Autodesk Inventor part; units mm, degrees
(part 8 of 11)
  line L1498 (15.1661, 13.0288) -> (15.4178, 12.4694)
  arc A2998 (15.3831, 12.4537) -> (15.4526, 12.485) centre (15.4178, 12.4694) ccw
  arc A2999 (15.2008, 13.0444) -> (15.1314, 13.0131) centre (15.1661, 13.0288) ccw
  line L1499 (15.4178, 12.4694) -> (15.6004, 11.8837)
  arc A3000 (15.5641, 11.8724) -> (15.6368, 11.8951) centre (15.6004, 11.8837) ccw
  arc A3001 (15.4542, 12.4807) -> (15.3815, 12.458) centre (15.4178, 12.4694) ccw
  line L1500 (15.6004, 11.8837) -> (15.7112, 11.2804)
  arc A3002 (15.6737, 11.2735) -> (15.7486, 11.2872) centre (15.7112, 11.2804) ccw
  arc A3003 (15.6379, 11.8906) -> (15.5629, 11.8769) centre (15.6004, 11.8837) ccw
  line L1501 (15.7112, 11.2804) -> (15.748, 10.668)
  arc A3004 (15.71, 10.6657) -> (15.786, 10.6703) centre (15.748, 10.668) ccw
  arc A3005 (15.7492, 11.2827) -> (15.6731, 11.2781) centre (15.7112, 11.2804) ccw
  line L1502 (15.748, 10.668) -> (15.6894, 10.0106)
  arc A3006 (15.6514, 10.014) -> (15.7273, 10.0072) centre (15.6894, 10.0106) ccw
  arc A3007 (15.7859, 10.6646) -> (15.71, 10.6714) centre (15.748, 10.668) ccw
  line L1503 (15.6894, 10.0106) -> (15.5482, 9.3659)
  arc A3008 (15.511, 9.3741) -> (15.5854, 9.3578) centre (15.5482, 9.3659) ccw
  arc A3009 (15.7266, 10.0025) -> (15.6522, 10.0188) centre (15.6894, 10.0106) ccw
  line L1504 (15.5482, 9.3659) -> (15.3268, 8.7442)
  arc A3010 (15.2909, 8.757) -> (15.3626, 8.7314) centre (15.3268, 8.7442) ccw
  arc A3011 (15.5841, 9.3532) -> (15.5123, 9.3787) centre (15.5482, 9.3659) ccw
  line L1505 (15.3268, 8.7442) -> (15.0285, 8.1555)
  arc A3012 (14.9945, 8.1727) -> (15.0625, 8.1383) centre (15.0285, 8.1555) ccw
  arc A3013 (15.3607, 8.727) -> (15.2928, 8.7614) centre (15.3268, 8.7442) ccw
  line L1506 (15.0285, 8.1555) -> (14.6584, 7.6091)
  arc A3014 (14.6268, 7.6305) -> (14.6899, 7.5877) centre (14.6584, 7.6091) ccw
  arc A3015 (15.0601, 8.1341) -> (14.997, 8.1768) centre (15.0285, 8.1555) ccw
  line L1507 (14.6584, 7.6091) -> (14.2222, 7.1138)
  arc A3016 (14.1936, 7.139) -> (14.2507, 7.0887) centre (14.2222, 7.1138) ccw
  arc A3017 (14.687, 7.5839) -> (14.6298, 7.6343) centre (14.6584, 7.6091) ccw
  line L1508 (14.2222, 7.1138) -> (13.7269, 6.6776)
  arc A3018 (13.7017, 6.7062) -> (13.7521, 6.649) centre (13.7269, 6.6776) ccw
  arc A3019 (14.2473, 7.0853) -> (14.197, 7.1424) centre (14.2222, 7.1138) ccw
  line L1509 (13.7269, 6.6776) -> (13.1805, 6.3075)
  arc A3020 (13.1592, 6.339) -> (13.2019, 6.2759) centre (13.1805, 6.3075) ccw
  arc A3021 (13.7483, 6.6461) -> (13.7055, 6.7092) centre (13.7269, 6.6776) ccw
  line L1510 (13.1805, 6.3075) -> (12.5917, 6.0093)
  arc A3022 (12.5745, 6.0433) -> (12.609, 5.9753) centre (12.5917, 6.0093) ccw
  arc A3023 (13.1977, 6.2735) -> (13.1633, 6.3415) centre (13.1805, 6.3075) ccw
  line L1511 (12.5917, 6.0093) -> (11.97, 5.7878)
  arc A3024 (11.9573, 5.8237) -> (11.9828, 5.7519) centre (11.97, 5.7878) ccw
  arc A3025 (12.6045, 5.9734) -> (12.579, 6.0452) centre (12.5917, 6.0093) ccw
  line L1512 (11.97, 5.7878) -> (11.3254, 5.6466)
  arc A3026 (11.3172, 5.6838) -> (11.3335, 5.6094) centre (11.3254, 5.6466) ccw
  arc A3027 (11.9782, 5.7506) -> (11.9619, 5.825) centre (11.97, 5.7878) ccw
  line L1513 (11.3254, 5.6466) -> (10.668, 5.588)
  arc A3028 (10.6646, 5.626) -> (10.6714, 5.5501) centre (10.668, 5.588) ccw
  arc A3029 (11.3288, 5.6087) -> (11.322, 5.6846) centre (11.3254, 5.6466) ccw
  line L1514 (10.668, 5.588) -> (10.668, 6.858)
  arc A3030 (10.7061, 6.858) -> (10.6299, 6.858) centre (10.668, 6.858) ccw
  arc A3031 (10.6299, 5.588) -> (10.7061, 5.588) centre (10.668, 5.588) ccw
  line L1515 (10.668, 6.858) -> (11.1934, 6.8774)
  arc A3032 (11.1948, 6.8393) -> (11.192, 6.9155) centre (11.1934, 6.8774) ccw
  arc A3033 (10.6666, 6.8961) -> (10.6694, 6.8199) centre (10.668, 6.858) ccw
  line L1516 (11.1934, 6.8774) -> (11.7108, 6.9714)
  arc A3034 (11.7176, 6.9339) -> (11.704, 7.0089) centre (11.7108, 6.9714) ccw
  arc A3035 (11.1866, 6.9149) -> (11.2003, 6.8399) centre (11.1934, 6.8774) ccw
  line L1517 (11.7108, 6.9714) -> (12.2094, 7.1381)
  arc A3036 (12.2215, 7.1019) -> (12.1974, 7.1742) centre (12.2094, 7.1381) ccw
  arc A3037 (11.6987, 7.0075) -> (11.7228, 6.9353) centre (11.7108, 6.9714) ccw
  line L1518 (12.2094, 7.1381) -> (12.6793, 7.374)
  arc A3038 (12.6964, 7.34) -> (12.6623, 7.4081) centre (12.6794, 7.374) ccw
  arc A3039 (12.1924, 7.1721) -> (12.2265, 7.104) centre (12.2094, 7.1381) ccw
  line L1519 (12.6793, 7.374) -> (13.1109, 7.6744)
  arc A3040 (13.1326, 7.6431) -> (13.0891, 7.7057) centre (13.1109, 7.6744) ccw
  arc A3041 (12.6576, 7.4053) -> (12.7011, 7.3427) centre (12.6793, 7.374) ccw
  line L1520 (13.1109, 7.6744) -> (13.4952, 8.0332)
  arc A3042 (13.5212, 8.0053) -> (13.4693, 8.061) centre (13.4952, 8.0332) ccw
  arc A3043 (13.0849, 7.7023) -> (13.1369, 7.6465) centre (13.1109, 7.6744) ccw
  line L1521 (13.4952, 8.0332) -> (13.8247, 8.443)
  arc A3044 (13.8544, 8.4191) -> (13.795, 8.4669) centre (13.8247, 8.443) ccw
  arc A3045 (13.4655, 8.057) -> (13.5249, 8.0093) centre (13.4952, 8.0332) ccw
  line L1522 (13.8247, 8.443) -> (14.0924, 8.8955)
  arc A3046 (14.1252, 8.8761) -> (14.0596, 8.9149) centre (14.0924, 8.8955) ccw
  arc A3047 (13.7919, 8.4624) -> (13.8575, 8.4236) centre (13.8247, 8.443) ccw
  line L1523 (14.0924, 8.8955) -> (14.293, 9.3815)
  arc A3048 (14.3282, 9.367) -> (14.2578, 9.3961) centre (14.293, 9.3815) ccw
  arc A3049 (14.0572, 8.91) -> (14.1276, 8.881) centre (14.0924, 8.8955) ccw
  line L1524 (14.293, 9.3815) -> (14.4224, 9.8911)
  arc A3050 (14.4594, 9.8818) -> (14.3855, 9.9005) centre (14.4224, 9.8911) ccw
  arc A3051 (14.2561, 9.3909) -> (14.33, 9.3721) centre (14.293, 9.3815) ccw
  line L1525 (14.4224, 9.8911) -> (14.478, 10.414)
  arc A3052 (14.5159, 10.41) -> (14.4401, 10.418) centre (14.478, 10.414) ccw
  arc A3053 (14.3845, 9.8952) -> (14.4603, 9.8871) centre (14.4224, 9.8911) ccw
  line L1526 (14.478, 10.414) -> (14.478, 10.668)
  arc A3054 (14.5161, 10.668) -> (14.4399, 10.668) centre (14.478, 10.668) ccw
  arc A3055 (14.4399, 10.414) -> (14.5161, 10.414) centre (14.478, 10.414) ccw
  line L1527 (14.478, 10.668) -> (14.4392, 11.2102)
  arc A3056 (14.4772, 11.2129) -> (14.4012, 11.2075) centre (14.4392, 11.2102) ccw
  arc A3057 (14.44, 10.6653) -> (14.516, 10.6707) centre (14.478, 10.668) ccw
  line L1528 (14.4392, 11.2102) -> (14.3237, 11.7414)
  arc A3058 (14.3609, 11.7495) -> (14.2864, 11.7333) centre (14.3237, 11.7414) ccw
  arc A3059 (14.402, 11.2021) -> (14.4764, 11.2183) centre (14.4392, 11.2102) ccw
  line L1529 (14.3237, 11.7414) -> (14.1337, 12.2507)
  arc A3060 (14.1694, 12.264) -> (14.098, 12.2374) centre (14.1337, 12.2507) ccw
  arc A3061 (14.288, 11.7281) -> (14.3594, 11.7547) centre (14.3237, 11.7414) ccw
  line L1530 (14.1337, 12.2507) -> (13.8732, 12.7278)
  arc A3062 (13.9066, 12.7461) -> (13.8397, 12.7096) centre (13.8732, 12.7278) ccw
  arc A3063 (14.1003, 12.2325) -> (14.1671, 12.269) centre (14.1337, 12.2507) ccw
  line L1531 (13.8732, 12.7278) -> (13.5474, 13.163)
  arc A3064 (13.5779, 13.1859) -> (13.5169, 13.1402) centre (13.5474, 13.163) ccw
  arc A3065 (13.8427, 12.705) -> (13.9037, 12.7507) centre (13.8732, 12.7278) ccw
  line L1532 (13.5474, 13.163) -> (13.163, 13.5474)
  arc A3066 (13.19, 13.5743) -> (13.1361, 13.5205) centre (13.163, 13.5474) ccw
  arc A3067 (13.5205, 13.1361) -> (13.5743, 13.19) centre (13.5474, 13.163) ccw
  line L1533 (13.163, 13.5474) -> (12.7278, 13.8732)
  arc A3068 (12.7507, 13.9037) -> (12.705, 13.8427) centre (12.7278, 13.8732) ccw
  arc A3069 (13.1402, 13.5169) -> (13.1859, 13.5779) centre (13.163, 13.5474) ccw
  line L1534 (12.7278, 13.8732) -> (12.2507, 14.1337)
  arc A3070 (12.269, 14.1671) -> (12.2325, 14.1003) centre (12.2507, 14.1337) ccw
  arc A3071 (12.7096, 13.8397) -> (12.7461, 13.9066) centre (12.7278, 13.8732) ccw
  line L1535 (12.2507, 14.1337) -> (11.7414, 14.3237)
  arc A3072 (11.7547, 14.3594) -> (11.7281, 14.288) centre (11.7414, 14.3237) ccw
  arc A3073 (12.2374, 14.098) -> (12.264, 14.1694) centre (12.2507, 14.1337) ccw
  line L1536 (11.7414, 14.3237) -> (11.2102, 14.4392)
  arc A3074 (11.2183, 14.4764) -> (11.2021, 14.402) centre (11.2102, 14.4392) ccw
  arc A3075 (11.7333, 14.2864) -> (11.7495, 14.3609) centre (11.7414, 14.3237) ccw
  line L1537 (11.2102, 14.4392) -> (10.668, 14.478)
  arc A3076 (10.6707, 14.516) -> (10.6653, 14.44) centre (10.668, 14.478) ccw
  arc A3077 (11.2075, 14.4012) -> (11.2129, 14.4772) centre (11.2102, 14.4392) ccw
  line L1538 (10.668, 14.478) -> (10.1258, 14.4392)
  arc A3078 (10.1231, 14.4772) -> (10.1285, 14.4012) centre (10.1258, 14.4392) ccw
  arc A3079 (10.6707, 14.44) -> (10.6653, 14.516) centre (10.668, 14.478) ccw
  line L1539 (10.1258, 14.4392) -> (9.5946, 14.3237)
  arc A3080 (9.5865, 14.3609) -> (9.6027, 14.2864) centre (9.5946, 14.3237) ccw
  arc A3081 (10.1339, 14.402) -> (10.1177, 14.4764) centre (10.1258, 14.4392) ccw
  line L1540 (9.5946, 14.3237) -> (9.0853, 14.1337)
  arc A3082 (9.072, 14.1694) -> (9.0986, 14.098) centre (9.0853, 14.1337) ccw
  arc A3083 (9.6079, 14.288) -> (9.5813, 14.3593) centre (9.5946, 14.3237) ccw
  line L1541 (9.0853, 14.1337) -> (8.6082, 13.8732)
  arc A3084 (8.5899, 13.9066) -> (8.6264, 13.8397) centre (8.6082, 13.8732) ccw
  arc A3085 (9.1035, 14.1003) -> (9.067, 14.1671) centre (9.0853, 14.1337) ccw
  line L1542 (8.6082, 13.8732) -> (8.173, 13.5474)
  arc A3086 (8.1501, 13.5779) -> (8.1958, 13.5169) centre (8.173, 13.5474) ccw
  arc A3087 (8.631, 13.8427) -> (8.5853, 13.9037) centre (8.6082, 13.8732) ccw
  line L1543 (8.173, 13.5474) -> (7.7886, 13.163)
  arc A3088 (7.7617, 13.19) -> (7.8155, 13.1361) centre (7.7886, 13.163) ccw
  arc A3089 (8.1999, 13.5205) -> (8.146, 13.5743) centre (8.173, 13.5474) ccw
  line L1544 (7.7886, 13.163) -> (7.4628, 12.7278)
  arc A3090 (7.4323, 12.7507) -> (7.4933, 12.705) centre (7.4628, 12.7278) ccw
  arc A3091 (7.8191, 13.1402) -> (7.7581, 13.1859) centre (7.7886, 13.163) ccw
  line L1545 (7.4628, 12.7278) -> (7.2023, 12.2507)
  arc A3092 (7.1689, 12.269) -> (7.2357, 12.2325) centre (7.2023, 12.2507) ccw
  arc A3093 (7.4963, 12.7096) -> (7.4294, 12.7461) centre (7.4628, 12.7278) ccw
  line L1546 (7.2023, 12.2507) -> (7.0123, 11.7414)
  arc A3094 (6.9766, 11.7547) -> (7.048, 11.7281) centre (7.0123, 11.7414) ccw
  arc A3095 (7.238, 12.2374) -> (7.1666, 12.264) centre (7.2023, 12.2507) ccw
  line L1547 (7.0123, 11.7414) -> (6.8968, 11.2102)
  arc A3096 (6.8596, 11.2183) -> (6.934, 11.2021) centre (6.8968, 11.2102) ccw
  arc A3097 (7.0496, 11.7333) -> (6.9751, 11.7495) centre (7.0123, 11.7414) ccw
  line L1548 (6.8968, 11.2102) -> (6.858, 10.668)
  arc A3098 (6.82, 10.6707) -> (6.896, 10.6653) centre (6.858, 10.668) ccw
  arc A3099 (6.9348, 11.2075) -> (6.8588, 11.2129) centre (6.8968, 11.2102) ccw
  line L1549 (6.858, 10.668) -> (6.8782, 10.1815)
  arc A3100 (6.8402, 10.18) -> (6.9163, 10.1831) centre (6.8782, 10.1815) ccw
  arc A3101 (6.8961, 10.6696) -> (6.8199, 10.6664) centre (6.858, 10.668) ccw
  line L1550 (6.8782, 10.1815) -> (6.9618, 9.7019)
  arc A3102 (6.9242, 9.6953) -> (6.9993, 9.7084) centre (6.9618, 9.7019) ccw
  arc A3103 (6.9158, 10.1881) -> (6.8407, 10.175) centre (6.8782, 10.1815) ccw
  line L1551 (6.9618, 9.7019) -> (7.1072, 9.2372)
  arc A3104 (7.0709, 9.2258) -> (7.1436, 9.2486) centre (7.1072, 9.2372) ccw
  arc A3105 (6.9982, 9.7133) -> (6.9254, 9.6905) centre (6.9618, 9.7019) ccw
  line L1552 (7.1072, 9.2372) -> (7.3121, 8.7955)
  arc A3106 (7.2775, 8.7795) -> (7.3466, 8.8116) centre (7.3121, 8.7955) ccw
  arc A3107 (7.1418, 9.2533) -> (7.0727, 9.2212) centre (7.1072, 9.2372) ccw
  line L1553 (7.3121, 8.7955) -> (7.5728, 8.3843)
  arc A3108 (7.5407, 8.364) -> (7.605, 8.4047) centre (7.5728, 8.3843) ccw
  arc A3109 (7.3443, 8.8159) -> (7.2799, 8.7751) centre (7.3121, 8.7955) ccw
  line L1554 (7.5728, 8.3843) -> (7.885, 8.0107)
  arc A3110 (7.8558, 7.9863) -> (7.9143, 8.0352) centre (7.885, 8.0107) ccw
  arc A3111 (7.6021, 8.4088) -> (7.5436, 8.3599) centre (7.5728, 8.3843) ccw
  line L1555 (7.885, 8.0107) -> (8.2433, 7.6811)
  arc A3112 (8.2175, 7.653) -> (8.2691, 7.7091) centre (8.2433, 7.6811) ccw
  arc A3113 (7.9108, 8.0388) -> (7.8592, 7.9827) centre (7.885, 8.0107) ccw
  line L1556 (8.2433, 7.6811) -> (8.6416, 7.401)
  arc A3114 (8.6196, 7.3698) -> (8.6635, 7.4321) centre (8.6416, 7.401) ccw
  arc A3115 (8.2652, 7.7122) -> (8.2214, 7.6499) centre (8.2433, 7.6811) ccw
  line L1557 (8.6416, 7.401) -> (9.073, 7.1753)
  arc A3116 (9.0553, 7.1415) -> (9.0906, 7.209) centre (9.073, 7.1753) ccw
  arc A3117 (8.6592, 7.4347) -> (8.6239, 7.3672) centre (8.6416, 7.401) ccw
  line L1558 (9.073, 7.1753) -> (9.27, 7.6205)
  arc A3118 (9.517, 6.972) -> (9.5432, 7.0436) centre (9.5301, 7.0078) ccw
  arc A3119 (9.0861, 7.211) -> (9.0599, 7.1395) centre (9.073, 7.1753) ccw
  line L1559 (9.27, 7.6205) -> (9.4072, 8.0877)
  arc A3120 (9.3988, 8.0505) -> (9.4155, 8.1249) centre (9.4072, 8.0877) ccw
  arc A3121 (9.2783, 7.6577) -> (9.2616, 7.5833) centre (9.27, 7.6205) ccw
  line L1560 (9.4072, 8.0877) -> (10.4902, 6.858)
  arc A3122 (10.4868, 6.8201) -> (10.4936, 6.896) centre (10.4902, 6.858) ccw
  arc A3123 (9.4106, 8.1256) -> (9.4038, 8.0497) centre (9.4072, 8.0877) ccw
  line L1561 (10.4902, 6.858) -> (10.4902, 5.588)
  arc A3124 (10.4521, 5.588) -> (10.5283, 5.588) centre (10.4902, 5.588) ccw
  arc A3125 (10.5283, 6.858) -> (10.4521, 6.858) centre (10.4902, 6.858) ccw
  line L1562 (9.9806, 15.6972) -> (11.3554, 15.6972)
  arc A3126 (11.3554, 15.6591) -> (11.3554, 15.7353) centre (11.3554, 15.6972) ccw
  arc A3127 (9.9806, 15.7353) -> (9.9806, 15.6591) centre (9.9806, 15.6972) ccw
  line L1563 (9.2739, 15.5448) -> (12.0621, 15.5448)
  arc A3128 (12.0621, 15.5067) -> (12.0621, 15.5829) centre (12.0621, 15.5448) ccw
  arc A3129 (9.2739, 15.5829) -> (9.2739, 15.5067) centre (9.2739, 15.5448) ccw
  line L1564 (8.81, 15.3924) -> (12.526, 15.3924)
  arc A3130 (12.526, 15.3543) -> (12.526, 15.4305) centre (12.526, 15.3924) ccw
  arc A3131 (8.81, 15.4305) -> (8.81, 15.3543) centre (8.81, 15.3924) ccw
  line L1565 (8.4714, 15.24) -> (12.8646, 15.24)
  arc A3132 (12.8646, 15.2019) -> (12.8646, 15.2781) centre (12.8646, 15.24) ccw
  arc A3133 (8.4714, 15.2781) -> (8.4714, 15.2019) centre (8.4714, 15.24) ccw
  line L1566 (8.1773, 15.0876) -> (13.1587, 15.0876)
  arc A3134 (13.1587, 15.0495) -> (13.1587, 15.1257) centre (13.1587, 15.0876) ccw
  arc A3135 (8.1773, 15.1257) -> (8.1773, 15.0495) centre (8.1773, 15.0876) ccw
  line L1567 (7.9252, 14.9352) -> (13.4108, 14.9352)
  arc A3136 (13.4108, 14.8971) -> (13.4108, 14.9733) centre (13.4108, 14.9352) ccw
  arc A3137 (7.9252, 14.9733) -> (7.9252, 14.8971) centre (7.9252, 14.9352) ccw
  line L1568 (7.698, 14.7828) -> (13.638, 14.7828)
  arc A3138 (13.638, 14.7447) -> (13.638, 14.8209) centre (13.638, 14.7828) ccw
  arc A3139 (7.698, 14.8209) -> (7.698, 14.7447) centre (7.698, 14.7828) ccw
  line L1569 (7.5035, 14.6304) -> (13.8325, 14.6304)
  arc A3140 (13.8325, 14.5923) -> (13.8325, 14.6685) centre (13.8325, 14.6304) ccw
  arc A3141 (7.5035, 14.6685) -> (7.5035, 14.5923) centre (7.5035, 14.6304) ccw
  line L1570 (7.309, 14.478) -> (10.668, 14.478)
  arc A3142 (10.668, 14.4399) -> (10.668, 14.5161) centre (10.668, 14.478) ccw
  arc A3143 (7.309, 14.5161) -> (7.309, 14.4399) centre (7.309, 14.478) ccw
  line L1571 (10.668, 14.478) -> (14.027, 14.478)
  arc A3144 (14.027, 14.4399) -> (14.027, 14.5161) centre (14.027, 14.478) ccw
  arc A3145 (10.668, 14.5161) -> (10.668, 14.4399) centre (10.668, 14.478) ccw
  line L1572 (7.1545, 14.3256) -> (9.6035, 14.3256)
  arc A3146 (9.6035, 14.2875) -> (9.6035, 14.3637) centre (9.6035, 14.3256) ccw
  arc A3147 (7.1545, 14.3637) -> (7.1545, 14.2875) centre (7.1545, 14.3256) ccw
  line L1573 (11.7325, 14.3256) -> (14.1815, 14.3256)
  arc A3148 (14.1815, 14.2875) -> (14.1815, 14.3637) centre (14.1815, 14.3256) ccw
  arc A3149 (11.7325, 14.3637) -> (11.7325, 14.2875) centre (11.7325, 14.3256) ccw
  line L1574 (7.0021, 14.1732) -> (9.1912, 14.1732)
  arc A3150 (9.1912, 14.1351) -> (9.1912, 14.2113) centre (9.1912, 14.1732) ccw
  arc A3151 (7.0021, 14.2113) -> (7.0021, 14.1351) centre (7.0021, 14.1732) ccw
  line L1575 (12.1448, 14.1732) -> (14.3339, 14.1732)
  arc A3152 (14.3339, 14.1351) -> (14.3339, 14.2113) centre (14.3339, 14.1732) ccw
  arc A3153 (12.1448, 14.2113) -> (12.1448, 14.1351) centre (12.1448, 14.1732) ccw
  line L1576 (6.8532, 14.0208) -> (8.8785, 14.0208)
  arc A3154 (8.8785, 13.9827) -> (8.8785, 14.0589) centre (8.8785, 14.0208) ccw
  arc A3155 (6.8532, 14.0589) -> (6.8532, 13.9827) centre (6.8532, 14.0208) ccw
  line L1577 (12.4575, 14.0208) -> (14.4829, 14.0208)
  arc A3156 (14.4829, 13.9827) -> (14.4829, 14.0589) centre (14.4829, 14.0208) ccw
  arc A3157 (12.4575, 14.0589) -> (12.4575, 13.9827) centre (12.4575, 14.0208) ccw
  line L1578 (6.7337, 13.8684) -> (8.6018, 13.8684)
  arc A3158 (8.6018, 13.8303) -> (8.6018, 13.9065) centre (8.6018, 13.8684) ccw
  arc A3159 (6.7337, 13.9065) -> (6.7337, 13.8303) centre (6.7337, 13.8684) ccw
  line L1579 (12.7342, 13.8684) -> (14.6023, 13.8684)
  arc A3160 (14.6023, 13.8303) -> (14.6023, 13.9065) centre (14.6023, 13.8684) ccw
  arc A3161 (12.7342, 13.9065) -> (12.7342, 13.8303) centre (12.7342, 13.8684) ccw
  line L1580 (6.6143, 13.716) -> (8.3982, 13.716)
  arc A3162 (8.3982, 13.6779) -> (8.3982, 13.7541) centre (8.3982, 13.716) ccw
  arc A3163 (6.6143, 13.7541) -> (6.6143, 13.6779) centre (6.6143, 13.716) ccw
  line L1581 (12.9378, 13.716) -> (14.7217, 13.716)
  arc A3164 (14.7217, 13.6779) -> (14.7217, 13.7541) centre (14.7217, 13.716) ccw
  arc A3165 (12.9378, 13.7541) -> (12.9378, 13.6779) centre (12.9378, 13.716) ccw
  line L1582 (6.4949, 13.5636) -> (8.1946, 13.5636)
  arc A3166 (8.1946, 13.5255) -> (8.1946, 13.6017) centre (8.1946, 13.5636) ccw
  arc A3167 (6.4949, 13.6017) -> (6.4949, 13.5255) centre (6.4949, 13.5636) ccw
  line L1583 (13.1414, 13.5636) -> (14.8411, 13.5636)
  arc A3168 (14.8411, 13.5255) -> (14.8411, 13.6017) centre (14.8411, 13.5636) ccw
  arc A3169 (13.1414, 13.6017) -> (13.1414, 13.5255) centre (13.1414, 13.5636) ccw
  line L1584 (6.4011, 13.4112) -> (8.0368, 13.4112)
  arc A3170 (8.0368, 13.3731) -> (8.0368, 13.4493) centre (8.0368, 13.4112) ccw
  arc A3171 (6.4011, 13.4493) -> (6.4011, 13.3731) centre (6.4011, 13.4112) ccw
  line L1585 (13.2992, 13.4113) -> (14.935, 13.4112)
  arc A3172 (14.935, 13.3731) -> (14.935, 13.4493) centre (14.935, 13.4112) ccw
  arc A3173 (13.2992, 13.4494) -> (13.2992, 13.3732) centre (13.2992, 13.4113) ccw
  line L1586 (6.3089, 13.2588) -> (7.8844, 13.2588)
  arc A3174 (7.8844, 13.2207) -> (7.8844, 13.2969) centre (7.8844, 13.2588) ccw
  arc A3175 (6.3089, 13.2969) -> (6.3089, 13.2207) centre (6.3089, 13.2588) ccw
  line L1587 (13.4516, 13.2589) -> (15.0271, 13.2588)
  arc A3176 (15.0271, 13.2207) -> (15.0271, 13.2969) centre (15.0271, 13.2588) ccw
  arc A3177 (13.4516, 13.297) -> (13.4516, 13.2208) centre (13.4516, 13.2589) ccw
  line L1588 (6.2168, 13.1064) -> (7.7463, 13.1064)
  arc A3178 (7.7463, 13.0683) -> (7.7463, 13.1445) centre (7.7463, 13.1064) ccw
  arc A3179 (6.2168, 13.1445) -> (6.2168, 13.0683) centre (6.2168, 13.1064) ccw
  line L1589 (13.5898, 13.1064) -> (15.1192, 13.1064)
  arc A3180 (15.1192, 13.0683) -> (15.1192, 13.1445) centre (15.1192, 13.1064) ccw
  arc A3181 (13.5898, 13.1445) -> (13.5898, 13.0683) centre (13.5898, 13.1064) ccw
  line L1590 (6.1362, 12.954) -> (7.6321, 12.954)
  arc A3182 (7.6321, 12.9159) -> (7.6321, 12.9921) centre (7.6321, 12.954) ccw
  arc A3183 (6.1362, 12.9921) -> (6.1362, 12.9159) centre (6.1362, 12.954) ccw
  line L1591 (13.7039, 12.9541) -> (15.1998, 12.954)
  arc A3184 (15.1998, 12.9159) -> (15.1998, 12.9921) centre (15.1998, 12.954) ccw
  arc A3185 (13.7039, 12.9922) -> (13.7039, 12.916) centre (13.7039, 12.9541) ccw
  line L1592 (6.0676, 12.8016) -> (7.5181, 12.8016)
  arc A3186 (7.5181, 12.7635) -> (7.5181, 12.8397) centre (7.5181, 12.8016) ccw
  arc A3187 (6.0676, 12.8397) -> (6.0676, 12.7635) centre (6.0676, 12.8016) ccw
  line L1593 (13.818, 12.8016) -> (15.2683, 12.8016)
  arc A3188 (15.2683, 12.7635) -> (15.2683, 12.8397) centre (15.2683, 12.8016) ccw
  arc A3189 (13.818, 12.8397) -> (13.818, 12.7635) centre (13.818, 12.8016) ccw
  line L1594 (5.9991, 12.6492) -> (7.4199, 12.6492)
  arc A3190 (7.4199, 12.6111) -> (7.4199, 12.6873) centre (7.4199, 12.6492) ccw
  arc A3191 (5.9991, 12.6873) -> (5.9991, 12.6111) centre (5.9991, 12.6492) ccw
  line L1595 (13.9161, 12.6492) -> (15.3369, 12.6492)
  arc A3192 (15.3369, 12.6111) -> (15.3369, 12.6873) centre (15.3369, 12.6492) ccw
  arc A3193 (13.9161, 12.6873) -> (13.9161, 12.6111) centre (13.9161, 12.6492) ccw
  line L1596 (5.9305, 12.4968) -> (7.3367, 12.4968)
  arc A3194 (7.3367, 12.4587) -> (7.3367, 12.5349) centre (7.3367, 12.4968) ccw
  arc A3195 (5.9305, 12.5349) -> (5.9305, 12.4587) centre (5.9305, 12.4968) ccw
  line L1597 (13.9993, 12.4968) -> (15.4055, 12.4968)
  arc A3196 (15.4055, 12.4587) -> (15.4055, 12.5349) centre (15.4055, 12.4968) ccw
  arc A3197 (13.9993, 12.5349) -> (13.9993, 12.4587) centre (13.9993, 12.4968) ccw
  line L1598 (5.8792, 12.3444) -> (7.2535, 12.3444)
  arc A3198 (7.2535, 12.3063) -> (7.2535, 12.3825) centre (7.2535, 12.3444) ccw
  arc A3199 (5.8792, 12.3825) -> (5.8792, 12.3063) centre (5.8792, 12.3444) ccw
  line L1599 (14.0825, 12.3444) -> (15.4568, 12.3444)
  arc A3200 (15.4568, 12.3063) -> (15.4568, 12.3825) centre (15.4568, 12.3444) ccw
  arc A3201 (14.0825, 12.3825) -> (14.0825, 12.3063) centre (14.0825, 12.3444) ccw
  line L1600 (5.8317, 12.192) -> (7.1804, 12.192)
  arc A3202 (7.1804, 12.1539) -> (7.1804, 12.2301) centre (7.1804, 12.192) ccw
  arc A3203 (5.8317, 12.2301) -> (5.8317, 12.1539) centre (5.8317, 12.192) ccw
  line L1601 (14.1556, 12.192) -> (15.5043, 12.192)
  arc A3204 (15.5043, 12.1539) -> (15.5043, 12.2301) centre (15.5043, 12.192) ccw
  arc A3205 (14.1556, 12.2301) -> (14.1556, 12.1539) centre (14.1556, 12.192) ccw
  line L1602 (5.7842, 12.0396) -> (7.1236, 12.0396)
  arc A3206 (7.1236, 12.0015) -> (7.1236, 12.0777) centre (7.1236, 12.0396) ccw
  arc A3207 (5.7842, 12.0777) -> (5.7842, 12.0015) centre (5.7842, 12.0396) ccw
  line L1603 (14.2124, 12.0396) -> (15.5518, 12.0396)
  arc A3208 (15.5518, 12.0015) -> (15.5518, 12.0777) centre (15.5518, 12.0396) ccw
  arc A3209 (14.2124, 12.0777) -> (14.2124, 12.0015) centre (14.2124, 12.0396) ccw
  line L1604 (5.7367, 11.8872) -> (7.0667, 11.8872)
  arc A3210 (7.0667, 11.8491) -> (7.0667, 11.9253) centre (7.0667, 11.8872) ccw
  arc A3211 (5.7367, 11.9253) -> (5.7367, 11.8491) centre (5.7367, 11.8872) ccw
  line L1605 (14.2693, 11.8872) -> (15.5993, 11.8872)
  arc A3212 (15.5993, 11.8491) -> (15.5993, 11.9253) centre (15.5993, 11.8872) ccw
  arc A3213 (14.2693, 11.9253) -> (14.2693, 11.8491) centre (14.2693, 11.8872) ccw
  line L1606 (5.7083, 11.7348) -> (7.0109, 11.7348)
  arc A3214 (7.0109, 11.6967) -> (7.0109, 11.7729) centre (7.0109, 11.7348) ccw
  arc A3215 (5.7083, 11.7729) -> (5.7083, 11.6967) centre (5.7083, 11.7348) ccw
  line L1607 (14.3251, 11.7348) -> (15.6277, 11.7348)
  arc A3216 (15.6277, 11.6967) -> (15.6277, 11.7729) centre (15.6277, 11.7348) ccw
  arc A3217 (14.3251, 11.7729) -> (14.3251, 11.6967) centre (14.3251, 11.7348) ccw
  line L1608 (5.6804, 11.5824) -> (6.9777, 11.5824)
  arc A3218 (6.9777, 11.5443) -> (6.9777, 11.6205) centre (6.9777, 11.5824) ccw
  arc A3219 (5.6804, 11.6205) -> (5.6804, 11.5443) centre (5.6804, 11.5824) ccw
  line L1609 (14.3583, 11.5824) -> (15.6557, 11.5824)
  arc A3220 (15.6557, 11.5443) -> (15.6557, 11.6205) centre (15.6557, 11.5824) ccw
  arc A3221 (14.3583, 11.6205) -> (14.3583, 11.5443) centre (14.3583, 11.5824) ccw
  line L1610 (5.6525, 11.43) -> (6.9446, 11.43)
  arc A3222 (6.9446, 11.3919) -> (6.9446, 11.4681) centre (6.9446, 11.43) ccw
  arc A3223 (5.6525, 11.4681) -> (5.6525, 11.3919) centre (5.6525, 11.43) ccw
  line L1611 (14.3914, 11.43) -> (15.6837, 11.43)
  arc A3224 (15.6837, 11.3919) -> (15.6837, 11.4681) centre (15.6837, 11.43) ccw
  arc A3225 (14.3914, 11.4681) -> (14.3914, 11.3919) centre (14.3914, 11.43) ccw
  line L1612 (5.6249, 11.2776) -> (6.9114, 11.2776)
  arc A3226 (6.9114, 11.2395) -> (6.9114, 11.3157) centre (6.9114, 11.2776) ccw
  arc A3227 (5.6249, 11.3157) -> (5.6249, 11.2395) centre (5.6249, 11.2776) ccw
  line L1613 (14.4246, 11.2776) -> (15.7111, 11.2776)
  arc A3228 (15.7111, 11.2395) -> (15.7111, 11.3157) centre (15.7111, 11.2776) ccw
  arc A3229 (14.4246, 11.3157) -> (14.4246, 11.2395) centre (14.4246, 11.2776) ccw
  line L1614 (5.6157, 11.1252) -> (6.8907, 11.1252)
  arc A3230 (6.8907, 11.0871) -> (6.8907, 11.1633) centre (6.8907, 11.1252) ccw
  arc A3231 (5.6157, 11.1633) -> (5.6157, 11.0871) centre (5.6157, 11.1252) ccw
  line L1615 (14.4455, 11.1257) -> (15.7205, 11.1252)
  arc A3232 (15.7205, 11.0871) -> (15.7205, 11.1633) centre (15.7205, 11.1252) ccw
  arc A3233 (14.4455, 11.1638) -> (14.4455, 11.0876) centre (14.4455, 11.1257) ccw
  line L1616 (5.6064, 10.9728) -> (6.8798, 10.9728)
  arc A3234 (6.8798, 10.9347) -> (6.8798, 11.0109) centre (6.8798, 10.9728) ccw
  arc A3235 (5.6064, 11.0109) -> (5.6064, 10.9347) centre (5.6064, 10.9728) ccw
  line L1617 (14.4562, 10.9728) -> (15.7297, 10.9728)
  arc A3236 (15.7297, 10.9347) -> (15.7297, 11.0109) centre (15.7297, 10.9728) ccw
  arc A3237 (14.4562, 11.0109) -> (14.4562, 10.9347) centre (14.4562, 10.9728) ccw
  line L1618 (5.5972, 10.8204) -> (6.8689, 10.8204)
  arc A3238 (6.8689, 10.7823) -> (6.8689, 10.8585) centre (6.8689, 10.8204) ccw
  arc A3239 (5.5972, 10.8585) -> (5.5972, 10.7823) centre (5.5972, 10.8204) ccw
  line L1619 (14.4671, 10.8204) -> (15.7388, 10.8204)
  arc A3240 (15.7388, 10.7823) -> (15.7388, 10.8585) centre (15.7388, 10.8204) ccw
  arc A3241 (14.4671, 10.8585) -> (14.4671, 10.7823) centre (14.4671, 10.8204) ccw
  line L1620 (5.588, 10.668) -> (6.858, 10.668)
  arc A3242 (6.858, 10.6299) -> (6.858, 10.7061) centre (6.858, 10.668) ccw
  arc A3243 (5.588, 10.7061) -> (5.588, 10.6299) centre (5.588, 10.668) ccw
  line L1621 (14.478, 10.668) -> (15.748, 10.668)
  arc A3244 (15.748, 10.6299) -> (15.748, 10.7061) centre (15.748, 10.668) ccw
  arc A3245 (14.478, 10.7061) -> (14.478, 10.6299) centre (14.478, 10.668) ccw
  line L1622 (5.5953, 10.5156) -> (6.8643, 10.5156)
  arc A3246 (6.8643, 10.4775) -> (6.8643, 10.5537) centre (6.8643, 10.5156) ccw
  arc A3247 (5.5953, 10.5537) -> (5.5953, 10.4775) centre (5.5953, 10.5156) ccw
  line L1623 (14.478, 10.5156) -> (15.7344, 10.5156)
  arc A3248 (15.7344, 10.4775) -> (15.7344, 10.5537) centre (15.7344, 10.5156) ccw
  arc A3249 (14.478, 10.5537) -> (14.478, 10.4775) centre (14.478, 10.5156) ccw
  line L1624 (5.6025, 10.3632) -> (6.8707, 10.3632)
  arc A3250 (6.8707, 10.3251) -> (6.8707, 10.4013) centre (6.8707, 10.3632) ccw
  arc A3251 (5.6025, 10.4013) -> (5.6025, 10.3251) centre (5.6025, 10.3632) ccw
  line L1625 (14.4726, 10.3632) -> (15.7208, 10.3632)
  arc A3252 (15.7208, 10.3251) -> (15.7208, 10.4013) centre (15.7208, 10.3632) ccw
  arc A3253 (14.4726, 10.4013) -> (14.4726, 10.3251) centre (14.4726, 10.3632) ccw
  line L1626 (5.6098, 10.2108) -> (6.877, 10.2108)
  arc A3254 (6.877, 10.1727) -> (6.877, 10.2489) centre (6.877, 10.2108) ccw
  arc A3255 (5.6098, 10.2489) -> (5.6098, 10.1727) centre (5.6098, 10.2108) ccw
  line L1627 (14.4564, 10.2108) -> (15.7072, 10.2108)
  arc A3256 (15.7072, 10.1727) -> (15.7072, 10.2489) centre (15.7072, 10.2108) ccw
  arc A3257 (14.4564, 10.2489) -> (14.4564, 10.1727) centre (14.4564, 10.2108) ccw
  line L1628 (5.6171, 10.0584) -> (6.8997, 10.0584)
  arc A3258 (6.8997, 10.0203) -> (6.8997, 10.0965) centre (6.8997, 10.0584) ccw
  arc A3259 (5.6171, 10.0965) -> (5.6171, 10.0203) centre (5.6171, 10.0584) ccw
  line L1629 (14.4402, 10.0584) -> (15.6936, 10.0584)
  arc A3260 (15.6936, 10.0203) -> (15.6936, 10.0965) centre (15.6936, 10.0584) ccw
  arc A3261 (14.4402, 10.0965) -> (14.4402, 10.0203) centre (14.4402, 10.0584) ccw
  line L1630 (5.6389, 9.906) -> (6.9262, 9.906)
  arc A3262 (6.9262, 9.8679) -> (6.9262, 9.9441) centre (6.9262, 9.906) ccw
  arc A3263 (5.6389, 9.9441) -> (5.6389, 9.8679) centre (5.6389, 9.906) ccw
  line L1631 (14.424, 9.906) -> (15.6665, 9.906)
  arc A3264 (15.6665, 9.8679) -> (15.6665, 9.9441) centre (15.6665, 9.906) ccw
  arc A3265 (14.424, 9.9441) -> (14.424, 9.8679) centre (14.424, 9.906) ccw
  line L1632 (5.6664, 9.7536) -> (6.9528, 9.7536)
  arc A3266 (6.9528, 9.7155) -> (6.9528, 9.7917) centre (6.9528, 9.7536) ccw
  arc A3267 (5.6664, 9.7917) -> (5.6664, 9.7155) centre (5.6664, 9.7536) ccw
  line L1633 (14.3875, 9.7536) -> (15.6331, 9.7536)
  arc A3268 (15.6331, 9.7155) -> (15.6331, 9.7917) centre (15.6331, 9.7536) ccw
  arc A3269 (14.3875, 9.7917) -> (14.3875, 9.7155) centre (14.3875, 9.7536) ccw
  line L1634 (5.6939, 9.6012) -> (6.9933, 9.6012)
  arc A3270 (6.9933, 9.5631) -> (6.9933, 9.6393) centre (6.9933, 9.6012) ccw
  arc A3271 (5.6939, 9.6393) -> (5.6939, 9.5631) centre (5.6939, 9.6012) ccw
  line L1635 (14.3488, 9.6012) -> (15.5997, 9.6012)
  arc A3272 (15.5997, 9.5631) -> (15.5997, 9.6393) centre (15.5997, 9.6012) ccw
  arc A3273 (14.3488, 9.6393) -> (14.3488, 9.5631) centre (14.3488, 9.6012) ccw
  line L1636 (5.7214, 9.4488) -> (7.041, 9.4488)
  arc A3274 (7.041, 9.4107) -> (7.041, 9.4869) centre (7.041, 9.4488) ccw
  arc A3275 (5.7214, 9.4869) -> (5.7214, 9.4107) centre (5.7214, 9.4488) ccw
  line L1637 (14.3101, 9.4488) -> (15.5663, 9.4488)
  arc A3276 (15.5663, 9.4107) -> (15.5663, 9.4869) centre (15.5663, 9.4488) ccw
  arc A3277 (14.3101, 9.4869) -> (14.3101, 9.4107) centre (14.3101, 9.4488) ccw
  line L1638 (5.7596, 9.2964) -> (7.0887, 9.2964)
  arc A3278 (7.0887, 9.2583) -> (7.0887, 9.3345) centre (7.0887, 9.2964) ccw
  arc A3279 (5.7596, 9.3345) -> (5.7596, 9.2583) centre (5.7596, 9.2964) ccw
  line L1639 (14.2579, 9.2964) -> (15.5234, 9.2964)
  arc A3280 (15.5234, 9.2583) -> (15.5234, 9.3345) centre (15.5234, 9.2964) ccw
  arc A3281 (14.2579, 9.3345) -> (14.2579, 9.2583) centre (14.2579, 9.2964) ccw
  line L1640 (5.8083, 9.144) -> (7.1505, 9.144)
  arc A3282 (7.1505, 9.1059) -> (7.1505, 9.1821) centre (7.1505, 9.144) ccw
  arc A3283 (5.8083, 9.1821) -> (5.8083, 9.1059) centre (5.8083, 9.144) ccw
  line L1641 (14.195, 9.144) -> (15.4691, 9.144)
  arc A3284 (15.4691, 9.1059) -> (15.4691, 9.1821) centre (15.4691, 9.144) ccw
  arc A3285 (14.195, 9.1821) -> (14.195, 9.1059) centre (14.195, 9.144) ccw
  line L1642 (5.8571, 8.9916) -> (7.2211, 8.9916)
  arc A3286 (7.2211, 8.9535) -> (7.2211, 9.0297) centre (7.2211, 8.9916) ccw
  arc A3287 (5.8571, 9.0297) -> (5.8571, 8.9535) centre (5.8571, 8.9916) ccw
  line L1643 (14.1321, 8.9916) -> (15.4149, 8.9916)
  arc A3288 (15.4149, 8.9535) -> (15.4149, 9.0297) centre (15.4149, 8.9916) ccw
  arc A3289 (14.1321, 9.0297) -> (14.1321, 8.9535) centre (14.1321, 8.9916) ccw
  line L1644 (5.9058, 8.8392) -> (7.2918, 8.8392)
  arc A3290 (7.2918, 8.8011) -> (7.2918, 8.8773) centre (7.2918, 8.8392) ccw
  arc A3291 (5.9058, 8.8773) -> (5.9058, 8.8011) centre (5.9058, 8.8392) ccw
  line L1645 (14.0591, 8.8392) -> (15.3606, 8.8392)
  arc A3292 (15.3606, 8.8011) -> (15.3606, 8.8773) centre (15.3606, 8.8392) ccw
  arc A3293 (14.0591, 8.8773) -> (14.0591, 8.8011) centre (14.0591, 8.8392) ccw
  line L1646 (5.9643, 8.6868) -> (7.381, 8.6868)
  arc A3294 (7.381, 8.6487) -> (7.381, 8.7249) centre (7.381, 8.6868) ccw
  arc A3295 (5.9643, 8.7249) -> (5.9643, 8.6487) centre (5.9643, 8.6868) ccw
  line L1647 (13.9689, 8.6868) -> (15.2977, 8.6868)
  arc A3296 (15.2977, 8.6487) -> (15.2977, 8.7249) centre (15.2977, 8.6868) ccw
  arc A3297 (13.9689, 8.7249) -> (13.9689, 8.6487) centre (13.9689, 8.6868) ccw
  line L1648 (6.0361, 8.5344) -> (7.4777, 8.5344)
  arc A3298 (7.4777, 8.4963) -> (7.4777, 8.5725) centre (7.4777, 8.5344) ccw
  arc A3299 (6.0361, 8.5725) -> (6.0361, 8.4963) centre (6.0361, 8.5344) ccw
  line L1649 (13.8788, 8.5344) -> (15.2204, 8.5344)
  arc A3300 (15.2204, 8.4963) -> (15.2204, 8.5725) centre (15.2204, 8.5344) ccw
  arc A3301 (13.8788, 8.5725) -> (13.8788, 8.4963) centre (13.8788, 8.5344) ccw
  line L1650 (6.1079, 8.382) -> (7.5748, 8.382)
  arc A3302 (7.5748, 8.3439) -> (7.5748, 8.4201) centre (7.5748, 8.382) ccw
  arc A3303 (6.1079, 8.4201) -> (6.1079, 8.3439) centre (6.1079, 8.382) ccw
  line L1651 (13.7757, 8.382) -> (15.1433, 8.382)
  arc A3304 (15.1433, 8.3439) -> (15.1433, 8.4201) centre (15.1433, 8.382) ccw
  arc A3305 (13.7757, 8.4201) -> (13.7757, 8.3439) centre (13.7757, 8.382) ccw
  line L1652 (6.1797, 8.2296) -> (7.7021, 8.2296)
  arc A3306 (7.7021, 8.1915) -> (7.7021, 8.2677) centre (7.7021, 8.2296) ccw
  arc A3307 (6.1797, 8.2677) -> (6.1797, 8.1915) centre (6.1797, 8.2296) ccw
  line L1653 (13.6531, 8.2296) -> (15.0661, 8.2296)
  arc A3308 (15.0661, 8.1915) -> (15.0661, 8.2677) centre (15.0661, 8.2296) ccw
  arc A3309 (13.6531, 8.2677) -> (13.6531, 8.1915) centre (13.6531, 8.2296) ccw
  line L1654 (6.2658, 8.0772) -> (7.8295, 8.0772)
  arc A3310 (7.8295, 8.0391) -> (7.8295, 8.1153) centre (7.8295, 8.0772) ccw
  arc A3311 (6.2658, 8.1153) -> (6.2658, 8.0391) centre (6.2658, 8.0772) ccw
  line L1655 (13.5306, 8.0772) -> (14.9755, 8.0772)
  arc A3312 (14.9755, 8.0391) -> (14.9755, 8.1153) centre (14.9755, 8.0772) ccw
  arc A3313 (13.5306, 8.1153) -> (13.5306, 8.0391) centre (13.5306, 8.0772) ccw
  line L1656 (6.3637, 7.9248) -> (7.9784, 7.9248)
  arc A3314 (7.9784, 7.8867) -> (7.9784, 7.9629) centre (7.9784, 7.9248) ccw
  arc A3315 (6.3637, 7.9629) -> (6.3637, 7.8867) centre (6.3637, 7.9248) ccw
  line L1657 (13.3791, 7.9248) -> (14.8723, 7.9248)
  arc A3316 (14.8723, 7.8867) -> (14.8723, 7.9629) centre (14.8723, 7.9248) ccw
  arc A3317 (13.3791, 7.9629) -> (13.3791, 7.8867) centre (13.3791, 7.9248) ccw
  line L1658 (6.4617, 7.7724) -> (8.144, 7.7724)
  arc A3318 (8.144, 7.7343) -> (8.144, 7.8105) centre (8.144, 7.7724) ccw
  arc A3319 (6.4617, 7.8105) -> (6.4617, 7.7343) centre (6.4617, 7.7724) ccw
  line L1659 (13.2159, 7.7724) -> (14.769, 7.7724)
  arc A3320 (14.769, 7.7343) -> (14.769, 7.8105) centre (14.769, 7.7724) ccw
  arc A3321 (13.2159, 7.8105) -> (13.2159, 7.7343) centre (13.2159, 7.7724) ccw
  line L1660 (6.5596, 7.62) -> (8.3301, 7.62)
  arc A3322 (8.3301, 7.5819) -> (8.3301, 7.6581) centre (8.3301, 7.62) ccw
  arc A3323 (6.5596, 7.6581) -> (6.5596, 7.5819) centre (6.5596, 7.62) ccw
  line L1661 (13.0327, 7.62) -> (14.6658, 7.62)
  arc A3324 (14.6658, 7.5819) -> (14.6658, 7.6581) centre (14.6658, 7.62) ccw
  arc A3325 (13.0327, 7.6581) -> (13.0327, 7.5819) centre (13.0327, 7.62) ccw
  line L1662 (6.6868, 7.4676) -> (8.5468, 7.4676)
  arc A3326 (8.5468, 7.4295) -> (8.5468, 7.5057) centre (8.5468, 7.4676) ccw
  arc A3327 (6.6868, 7.5057) -> (6.6868, 7.4295) centre (6.6868, 7.4676) ccw
  line L1663 (12.8138, 7.4676) -> (14.5337, 7.4676)
  arc A3328 (14.5337, 7.4295) -> (14.5337, 7.5057) centre (14.5337, 7.4676) ccw
  arc A3329 (12.8138, 7.5057) -> (12.8138, 7.4295) centre (12.8138, 7.4676) ccw
  line L1664 (6.8157, 7.3152) -> (8.8055, 7.3152)
  arc A3330 (8.8055, 7.2771) -> (8.8055, 7.3533) centre (8.8055, 7.3152) ccw
  arc A3331 (6.8157, 7.3533) -> (6.8157, 7.2771) centre (6.8157, 7.3152) ccw
  line L1665 (12.5622, 7.3152) -> (14.3995, 7.3152)
  arc A3332 (14.3995, 7.2771) -> (14.3995, 7.3533) centre (14.3995, 7.3152) ccw
  arc A3333 (12.5622, 7.3533) -> (12.5622, 7.2771) centre (12.5622, 7.3152) ccw
  line L1666 (6.9446, 7.1628) -> (9.0876, 7.2084)
  arc A3334 (9.0876, 7.1703) -> (9.0876, 7.2465) centre (9.0876, 7.2084) ccw
  arc A3335 (6.9446, 7.2009) -> (6.9446, 7.1247) centre (6.9446, 7.1628) ccw
  line L1667 (12.2587, 7.1628) -> (14.2653, 7.1628)
  arc A3336 (14.2653, 7.1247) -> (14.2653, 7.2009) centre (14.2653, 7.1628) ccw
  arc A3337 (12.2587, 7.2009) -> (12.2587, 7.1247) centre (12.2587, 7.1628) ccw
  line L1668 (7.0995, 7.0104) -> (9.2669, 7.6136)
  arc A3338 (9.2669, 7.5755) -> (9.2669, 7.6517) centre (9.2669, 7.6136) ccw
  arc A3339 (7.0995, 7.0485) -> (7.0995, 6.9723) centre (7.0995, 7.0104) ccw
  line L1669 (11.8274, 7.0104) -> (14.1047, 7.0104)
  arc A3340 (14.1047, 6.9723) -> (14.1047, 7.0485) centre (14.1047, 7.0104) ccw
  arc A3341 (11.8274, 7.0485) -> (11.8274, 6.9723) centre (11.8274, 7.0104) ccw
  line L1670 (7.2672, 6.858) -> (10.4902, 6.858)
  arc A3342 (10.4902, 6.8199) -> (10.4902, 6.8961) centre (10.4902, 6.858) ccw
  arc A3343 (7.2672, 6.8961) -> (7.2672, 6.8199) centre (7.2672, 6.858) ccw
  line L1671 (10.668, 6.858) -> (13.9317, 6.858)
  arc A3344 (13.9317, 6.8199) -> (13.9317, 6.8961) centre (13.9317, 6.858) ccw
  arc A3345 (10.668, 6.8961) -> (10.668, 6.8199) centre (10.668, 6.858) ccw
  line L1672 (7.4349, 6.7056) -> (10.4902, 6.7056)
  arc A3346 (10.4902, 6.6675) -> (10.4902, 6.7437) centre (10.4902, 6.7056) ccw
  arc A3347 (7.4349, 6.7437) -> (7.4349, 6.6675) centre (7.4349, 6.7056) ccw
  line L1673 (10.668, 6.7056) -> (13.7586, 6.7056)
  arc A3348 (13.7586, 6.6675) -> (13.7586, 6.7437) centre (13.7586, 6.7056) ccw
  arc A3349 (10.668, 6.7437) -> (10.668, 6.6675) centre (10.668, 6.7056) ccw
  line L1674 (7.6435, 6.5532) -> (10.4902, 6.5532)
  arc A3350 (10.4902, 6.5151) -> (10.4902, 6.5913) centre (10.4902, 6.5532) ccw
  arc A3351 (7.6435, 6.5913) -> (7.6435, 6.5151) centre (7.6435, 6.5532) ccw
  line L1675 (10.668, 6.5533) -> (13.5432, 6.5532)
  arc A3352 (13.5432, 6.5151) -> (13.5432, 6.5913) centre (13.5432, 6.5532) ccw
  arc A3353 (10.668, 6.5914) -> (10.668, 6.5152) centre (10.668, 6.5533) ccw
  line L1676 (7.863, 6.4008) -> (10.4902, 6.4008)
  arc A3354 (10.4902, 6.3627) -> (10.4902, 6.4389) centre (10.4902, 6.4008) ccw
  arc A3355 (7.863, 6.4389) -> (7.863, 6.3627) centre (7.863, 6.4008) ccw
  line L1677 (10.668, 6.4009) -> (13.3183, 6.4008)
  arc A3356 (13.3183, 6.3627) -> (13.3183, 6.4389) centre (13.3183, 6.4008) ccw
  arc A3357 (10.668, 6.439) -> (10.668, 6.3628) centre (10.668, 6.4009) ccw
  line L1678 (8.1088, 6.2484) -> (10.4902, 6.2484)
  arc A3358 (10.4902, 6.2103) -> (10.4902, 6.2865) centre (10.4902, 6.2484) ccw
  arc A3359 (8.1088, 6.2865) -> (8.1088, 6.2103) centre (8.1088, 6.2484) ccw
  line L1679 (10.668, 6.2484) -> (13.0639, 6.2484)
  arc A3360 (13.0639, 6.2103) -> (13.0639, 6.2865) centre (13.0639, 6.2484) ccw
  arc A3361 (10.668, 6.2865) -> (10.668, 6.2103) centre (10.668, 6.2484) ccw
  line L1680 (8.4045, 6.096) -> (10.4902, 6.096)
  arc A3362 (10.4902, 6.0579) -> (10.4902, 6.1341) centre (10.4902, 6.096) ccw
  arc A3363 (8.4045, 6.1341) -> (8.4045, 6.0579) centre (8.4045, 6.096) ccw
  line L1681 (10.668, 6.096) -> (12.763, 6.096)
  arc A3364 (12.763, 6.0579) -> (12.763, 6.1341) centre (12.763, 6.096) ccw
  arc A3365 (10.668, 6.1341) -> (10.668, 6.0579) centre (10.668, 6.096) ccw
  line L1682 (8.7493, 5.9436) -> (10.4902, 5.9436)
  arc A3366 (10.4902, 5.9055) -> (10.4902, 5.9817) centre (10.4902, 5.9436) ccw
  arc A3367 (8.7493, 5.9817) -> (8.7493, 5.9055) centre (8.7493, 5.9436) ccw
  line L1683 (10.668, 5.9436) -> (12.4074, 5.9436)
  arc A3368 (12.4074, 5.9055) -> (12.4074, 5.9817) centre (12.4074, 5.9436) ccw
  arc A3369 (10.668, 5.9817) -> (10.668, 5.9055) centre (10.668, 5.9436) ccw
  line L1684 (9.1733, 5.7912) -> (10.4902, 5.7912)
  arc A3370 (10.4902, 5.7531) -> (10.4902, 5.8293) centre (10.4902, 5.7912) ccw
  arc A3371 (9.1733, 5.8293) -> (9.1733, 5.7531) centre (9.1733, 5.7912) ccw
  line L1685 (10.668, 5.7912) -> (11.9796, 5.7912)
  arc A3372 (11.9796, 5.7531) -> (11.9796, 5.8293) centre (11.9796, 5.7912) ccw
  arc A3373 (10.668, 5.8293) -> (10.668, 5.7531) centre (10.668, 5.7912) ccw
  line L1686 (9.8815, 5.6388) -> (10.4902, 5.6388)
  arc A3374 (10.4902, 5.6007) -> (10.4902, 5.6769) centre (10.4902, 5.6388) ccw
  arc A3375 (9.8815, 5.6769) -> (9.8815, 5.6007) centre (9.8815, 5.6388) ccw
  line L1687 (10.668, 5.6388) -> (11.2376, 5.6388)
  arc A3376 (11.2376, 5.6007) -> (11.2376, 5.6769) centre (11.2376, 5.6388) ccw
  arc A3377 (10.668, 5.6769) -> (10.668, 5.6007) centre (10.668, 5.6388) ccw
  line L1688 (10.4902, 5.588) -> (9.8395, 5.6423)
  arc A3378 (9.8426, 5.6803) -> (9.8363, 5.6043) centre (9.8395, 5.6423) ccw
  arc A3379 (10.487, 5.55) -> (10.4934, 5.626) centre (10.4902, 5.588) ccw
  line L1689 (9.8395, 5.6423) -> (9.2014, 5.7811)
  arc A3380 (9.2095, 5.8183) -> (9.1933, 5.7439) centre (9.2014, 5.7811) ccw
  arc A3381 (9.8314, 5.6051) -> (9.8476, 5.6795) centre (9.8395, 5.6423) ccw
  line L1690 (9.2014, 5.7811) -> (8.5869, 6.0019)
  arc A3382 (8.5998, 6.0378) -> (8.5741, 5.9661) centre (8.5869, 6.002) ccw
  arc A3383 (9.1885, 5.7452) -> (9.2143, 5.8169) centre (9.2014, 5.7811) ccw
  line L1691 (8.5869, 6.0019) -> (8.0066, 6.3011)
  arc A3384 (8.024, 6.335) -> (7.9891, 6.2673) centre (8.0066, 6.3011) ccw
  arc A3385 (8.5695, 5.9681) -> (8.6044, 6.0358) centre (8.5869, 6.0019) ccw
  line L1692 (8.0066, 6.3011) -> (7.4702, 6.6735)
  arc A3386 (7.4919, 6.7048) -> (7.4484, 6.6422) centre (7.4702, 6.6735) ccw
  arc A3387 (7.9848, 6.2698) -> (8.0283, 6.3324) centre (8.0065, 6.3011) ccw
  line L1693 (7.4702, 6.6735) -> (6.987, 7.1127)
  arc A3388 (7.0126, 7.1409) -> (6.9614, 7.0845) centre (6.987, 7.1127) ccw
  arc A3389 (7.4446, 6.6453) -> (7.4958, 6.7017) centre (7.4702, 6.6735) ccw
  line L1694 (6.987, 7.1127) -> (6.5653, 7.6112)
  arc A3390 (6.5944, 7.6358) -> (6.5362, 7.5866) centre (6.5653, 7.6112) ccw
  arc A3391 (6.9579, 7.0881) -> (7.0161, 7.1373) centre (6.987, 7.1127) ccw
  line L1695 (6.5653, 7.6112) -> (6.2122, 8.1605)
  arc A3392 (6.2443, 8.1811) -> (6.1802, 8.1399) centre (6.2122, 8.1605) ccw
  arc A3393 (6.5332, 7.5906) -> (6.5973, 7.6318) centre (6.5653, 7.6112) ccw
  line L1696 (6.2122, 8.1605) -> (5.9339, 8.7512)
  arc A3394 (5.9684, 8.7675) -> (5.8994, 8.735) centre (5.9339, 8.7512) ccw
  arc A3395 (6.1778, 8.1443) -> (6.2467, 8.1768) centre (6.2122, 8.1605) ccw
  line L1697 (5.9339, 8.7512) -> (5.7351, 9.3732)
  arc A3396 (5.7714, 9.3848) -> (5.6988, 9.3616) centre (5.7351, 9.3732) ccw
  arc A3397 (5.8976, 8.7396) -> (5.9702, 8.7628) centre (5.9339, 8.7512) ccw
  line L1698 (5.7351, 9.3732) -> (5.6191, 10.0158)
  arc A3398 (5.6566, 10.0225) -> (5.5816, 10.009) centre (5.6191, 10.0158) ccw
  arc A3399 (5.6976, 9.3664) -> (5.7726, 9.3799) centre (5.7351, 9.3732) ccw
  line L1699 (5.6191, 10.0158) -> (5.588, 10.668)
  arc A3400 (5.6261, 10.6698) -> (5.55, 10.6662) centre (5.588, 10.668) ccw
  arc A3401 (5.581, 10.0139) -> (5.6572, 10.0176) centre (5.6191, 10.0158) ccw
  line L1700 (5.588, 10.668) -> (5.625, 11.2803)
  arc A3402 (5.6631, 11.278) -> (5.587, 11.2826) centre (5.625, 11.2803) ccw
  arc A3403 (5.55, 10.6703) -> (5.626, 10.6657) centre (5.588, 10.668) ccw
  line L1701 (5.625, 11.2803) -> (5.7356, 11.8837)
  arc A3404 (5.7731, 11.8769) -> (5.6981, 11.8906) centre (5.7356, 11.8837) ccw
  arc A3405 (5.5876, 11.2872) -> (5.6625, 11.2734) centre (5.625, 11.2803) ccw
  line L1702 (5.7356, 11.8837) -> (5.9181, 12.4694)
  arc A3406 (5.9545, 12.4581) -> (5.8818, 12.4807) centre (5.9181, 12.4694) ccw
  arc A3407 (5.6993, 11.895) -> (5.772, 11.8724) centre (5.7356, 11.8837) ccw
  line L1703 (5.9181, 12.4694) -> (6.1699, 13.0288)
  arc A3408 (6.2046, 13.0131) -> (6.1351, 13.0444) centre (6.1699, 13.0288) ccw
  arc A3409 (5.8834, 12.485) -> (5.9529, 12.4537) centre (5.9181, 12.4694) ccw
  line L1704 (6.1699, 13.0288) -> (6.4872, 13.5538)
  arc A3410 (6.5199, 13.534) -> (6.4546, 13.5735) centre (6.4872, 13.5538) ccw
  arc A3411 (6.1373, 13.0485) -> (6.2025, 13.0091) centre (6.1699, 13.0288) ccw
  line L1705 (6.4872, 13.5538) -> (6.8656, 14.0367)
  arc A3412 (6.8956, 14.0131) -> (6.8356, 14.0602) centre (6.8656, 14.0367) ccw
  arc A3413 (6.4572, 13.5773) -> (6.5172, 13.5303) centre (6.4872, 13.5538) ccw
  line L1706 (6.8656, 14.0367) -> (7.2993, 14.4704)
  arc A3414 (7.3263, 14.4435) -> (7.2724, 14.4974) centre (7.2993, 14.4704) ccw
  arc A3415 (6.8386, 14.0636) -> (6.8925, 14.0097) centre (6.8656, 14.0367) ccw
  line L1707 (7.2993, 14.4704) -> (7.7822, 14.8488)
  arc A3416 (7.8057, 14.8188) -> (7.7587, 14.8788) centre (7.7822, 14.8488) ccw
  arc A3417 (7.2758, 14.5004) -> (7.3228, 14.4404) centre (7.2993, 14.4704) ccw
  line L1708 (7.7822, 14.8488) -> (8.3072, 15.1661)
  arc A3418 (8.3269, 15.1335) -> (8.2875, 15.1987) centre (8.3072, 15.1661) ccw
  arc A3419 (7.7625, 14.8814) -> (7.8019, 14.8161) centre (7.7822, 14.8488) ccw
  line L1709 (8.3072, 15.1661) -> (8.8666, 15.4179)
  arc A3420 (8.8823, 15.3831) -> (8.851, 15.4526) centre (8.8666, 15.4179) ccw
  arc A3421 (8.2916, 15.2009) -> (8.3228, 15.1314) centre (8.3072, 15.1661) ccw
  line L1710 (8.8666, 15.4179) -> (9.4523, 15.6004)
  arc A3422 (9.4636, 15.564) -> (9.441, 15.6367) centre (9.4523, 15.6004) ccw
  arc A3423 (8.8553, 15.4542) -> (8.8779, 15.3815) centre (8.8666, 15.4179) ccw
  line L1711 (9.4523, 15.6004) -> (10.0557, 15.711)
  arc A3424 (10.0625, 15.6735) -> (10.0488, 15.7484) centre (10.0557, 15.7109) ccw
  arc A3425 (9.4454, 15.6379) -> (9.4591, 15.5629) centre (9.4523, 15.6004) ccw
  line L1712 (10.0557, 15.711) -> (10.668, 15.748)
  arc A3426 (10.6703, 15.71) -> (10.6657, 15.786) centre (10.668, 15.748) ccw
  arc A3427 (10.0534, 15.749) -> (10.058, 15.6729) centre (10.0557, 15.711) ccw
  line L1713 (10.668, 15.748) -> (11.2803, 15.711)
  arc A3428 (11.278, 15.6729) -> (11.2826, 15.749) centre (11.2803, 15.711) ccw
  arc A3429 (10.6703, 15.786) -> (10.6657, 15.71) centre (10.668, 15.748) ccw
  line L1714 (11.2803, 15.711) -> (11.8837, 15.6004)
  arc A3430 (11.8769, 15.5629) -> (11.8906, 15.6379) centre (11.8837, 15.6004) ccw
  arc A3431 (11.2872, 15.7484) -> (11.2735, 15.6735) centre (11.2803, 15.7109) ccw
  line L1715 (11.8837, 15.6004) -> (12.4694, 15.4179)
  arc A3432 (12.4581, 15.3815) -> (12.4807, 15.4542) centre (12.4694, 15.4179) ccw
  arc A3433 (11.8951, 15.6367) -> (11.8724, 15.564) centre (11.8837, 15.6004) ccw
  line L1716 (12.4694, 15.4179) -> (13.0288, 15.1661)
  arc A3434 (13.0132, 15.1313) -> (13.0444, 15.2008) centre (13.0288, 15.1661) ccw
  arc A3435 (12.485, 15.4526) -> (12.4538, 15.3831) centre (12.4694, 15.4179) ccw
  line L1717 (13.0288, 15.1661) -> (13.5538, 14.8487)
  arc A3436 (13.5341, 14.8161) -> (13.5735, 14.8814) centre (13.5538, 14.8487) ccw
  arc A3437 (13.0485, 15.1987) -> (13.0091, 15.1335) centre (13.0288, 15.1661) ccw
  line L1718 (13.5538, 14.8487) -> (14.0367, 14.4704)
  arc A3438 (14.0132, 14.4404) -> (14.0602, 14.5004) centre (14.0367, 14.4704) ccw
  arc A3439 (13.5773, 14.8787) -> (13.5303, 14.8187) centre (13.5538, 14.8487) ccw
  line L1719 (14.0367, 14.4704) -> (14.4704, 14.0367)
  arc A3440 (14.4435, 14.0097) -> (14.4974, 14.0636) centre (14.4704, 14.0367) ccw
  arc A3441 (14.0636, 14.4974) -> (14.0097, 14.4435) centre (14.0367, 14.4704) ccw
  line L1720 (14.4704, 14.0367) -> (14.8488, 13.5538)
  arc A3442 (14.8188, 13.5303) -> (14.8788, 13.5773) centre (14.8488, 13.5538) ccw
  arc A3443 (14.5004, 14.0602) -> (14.4405, 14.0132) centre (14.4704, 14.0367) ccw
  line L1721 (14.8488, 13.5538) -> (15.1661, 13.0288)
  arc A3444 (15.1335, 13.0091) -> (15.1987, 13.0485) centre (15.1661, 13.0288) ccw
  arc A3445 (14.8814, 13.5735) -> (14.8162, 13.5341) centre (14.8488, 13.5538) ccw
  line L1722 (15.1661, 13.0288) -> (15.4178, 12.4694)
  arc A3446 (15.3831, 12.4537) -> (15.4526, 12.485) centre (15.4178, 12.4694) ccw
  arc A3447 (15.2008, 13.0444) -> (15.1314, 13.0131) centre (15.1661, 13.0288) ccw
  line L1723 (15.4178, 12.4694) -> (15.6004, 11.8837)
  arc A3448 (15.5641, 11.8724) -> (15.6368, 11.8951) centre (15.6004, 11.8837) ccw
  arc A3449 (15.4542, 12.4807) -> (15.3815, 12.458) centre (15.4178, 12.4694) ccw
  line L1724 (15.6004, 11.8837) -> (15.7112, 11.2804)
  arc A3450 (15.6737, 11.2735) -> (15.7486, 11.2872) centre (15.7112, 11.2804) ccw
  arc A3451 (15.6379, 11.8906) -> (15.5629, 11.8769) centre (15.6004, 11.8837) ccw
  line L1725 (15.7112, 11.2804) -> (15.748, 10.668)
  arc A3452 (15.71, 10.6657) -> (15.786, 10.6703) centre (15.748, 10.668) ccw
  arc A3453 (15.7492, 11.2827) -> (15.6731, 11.2781) centre (15.7112, 11.2804) ccw
  line L1726 (15.748, 10.668) -> (15.6894, 10.0106)
  arc A3454 (15.6514, 10.014) -> (15.7273, 10.0072) centre (15.6894, 10.0106) ccw
  arc A3455 (15.7859, 10.6646) -> (15.71, 10.6714) centre (15.748, 10.668) ccw
  line L1727 (15.6894, 10.0106) -> (15.5482, 9.3659)
  arc A3456 (15.511, 9.3741) -> (15.5854, 9.3578) centre (15.5482, 9.3659) ccw
  arc A3457 (15.7266, 10.0025) -> (15.6522, 10.0188) centre (15.6894, 10.0106) ccw
  line L1728 (15.5482, 9.3659) -> (15.3268, 8.7442)
  arc A3458 (15.2909, 8.757) -> (15.3626, 8.7314) centre (15.3268, 8.7442) ccw
  arc A3459 (15.5841, 9.3532) -> (15.5123, 9.3787) centre (15.5482, 9.3659) ccw
  line L1729 (15.3268, 8.7442) -> (15.0285, 8.1555)
  arc A3460 (14.9945, 8.1727) -> (15.0625, 8.1383) centre (15.0285, 8.1555) ccw
  arc A3461 (15.3607, 8.727) -> (15.2928, 8.7614) centre (15.3268, 8.7442) ccw
  line L1730 (15.0285, 8.1555) -> (14.6584, 7.6091)
  arc A3462 (14.6268, 7.6305) -> (14.6899, 7.5877) centre (14.6584, 7.6091) ccw
  arc A3463 (15.0601, 8.1341) -> (14.997, 8.1768) centre (15.0285, 8.1555) ccw
  line L1731 (14.6584, 7.6091) -> (14.2222, 7.1138)
  arc A3464 (14.1936, 7.139) -> (14.2507, 7.0887) centre (14.2222, 7.1138) ccw
  arc A3465 (14.687, 7.5839) -> (14.6298, 7.6343) centre (14.6584, 7.6091) ccw
  line L1732 (14.2222, 7.1138) -> (13.7269, 6.6776)
  arc A3466 (13.7017, 6.7062) -> (13.7521, 6.649) centre (13.7269, 6.6776) ccw
  arc A3467 (14.2473, 7.0853) -> (14.197, 7.1424) centre (14.2222, 7.1138) ccw
  line L1733 (13.7269, 6.6776) -> (13.1805, 6.3075)
  arc A3468 (13.1592, 6.339) -> (13.2019, 6.2759) centre (13.1805, 6.3075) ccw
  arc A3469 (13.7483, 6.6461) -> (13.7055, 6.7092) centre (13.7269, 6.6776) ccw
  line L1734 (13.1805, 6.3075) -> (12.5917, 6.0093)
  arc A3470 (12.5745, 6.0433) -> (12.609, 5.9753) centre (12.5917, 6.0093) ccw
  arc A3471 (13.1977, 6.2735) -> (13.1633, 6.3415) centre (13.1805, 6.3075) ccw